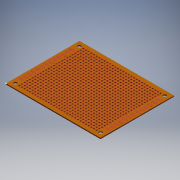
# Autodesk Inventor part: Adafruit_ProtoBoard
Saved by Autodesk Inventor 2018 (Build 220112000, 112)
## iProperties
Created: 2019-08-07
Part Number: Adafruit_ProtoBoard
Material: Generic
Document SubType Name: Modeling
Designer: jhernandez
Density: 1 g/cm^3
Appearance: Copper - Polished
Author: jhernandez
Autodesk Inventor part; units mm, degrees
(part 1 of 4)
ref_plane "YZ Plane" through (0, 0, 0) normal (1, 0, 0) x (0, 1, 0)
ref_plane "XZ Plane" through (0, 0, 0) normal (0, 1, 0) x (-1, 0, 0)
ref_plane "XY Plane" through (0, 0, 0) normal (0, 0, 1) x (1, 0, 0)
sketch "Sketch1" plane through (0, 0, 0) normal (0, 1, 0) x (-1, 0, 0)
  line L0 (0, 0) -> (-90, 0)
  line L1 (-90, 0) -> (-90, -70)
  line L2 (-90, -70) -> (0, -70)
  line L3 (0, -70) -> (0, 0)
  dimension "d0" = 90
  dimension "d1" = 70
  constraints: 8 end point, 2 parallel, 1 horizontal, 1 perpendicular
  measures "d0" distance of L1.end L2.end
  measures "d1" distance of L0.end L1.end
extrude "Extrusion1" add sketch "Sketch1" along normal blind 1
sketch "Sketch2" plane through (0, 1, 0) normal (0, 1, 0) x (1, 0, 0)
  line L0 (0, 0) -> (90, 0) construction
  line L1 (90, 0) -> (90, 70) construction
  line L2 (90, 70) -> (0, 70) construction
  line L3 (0, 70) -> (0, 0) construction
  line L4 (0, 70) -> (0, 0) construction
  line L5 (0, 35) -> (90, 35) construction
  line L6 (90, 70) -> (0, 70) construction
  line L7 (45, 70) -> (45, 0) construction
  circle A0 centre (4.36, 65.48) radius 1.5494
  circle A1 centre (85.64, 65.48) radius 1.5494
  circle A2 centre (4.36, 4.52) radius 1.5494
  circle A3 centre (85.64, 4.52) radius 1.5494
  dimension "d4" = 81.28
  dimension "d5" = 60.96
  dimension "d6" = 3.0988
  constraints: 4 centre point, 4 end point, 4 midpoint, 3 symmetric about line, 3 other
  measures "d4" diameter of A0.centre L7
  measures "d5" diameter of A0.centre L5
  measures "d6" diameter of A0
extrude "Mounting_Holes" cut sketch "Sketch2" against normal up to next
sketch "Sketch5" plane through (0, 1, 0) normal (0, 1, 0) x (1, 0, 0)
  line L0 (90, 70) -> (0, 70) construction
  line L1 (90, 0) -> (90, 70) construction
  line L2 (0, 0) -> (90, 0) construction
  line L3 (0, 70) -> (0, 0) construction
  line L4 (90, 0) -> (90, 70) construction
  line L5 (90, 35) -> (0, 35) construction
  line L6 (45, 70) -> (45, 0) construction
  line L7 (87.4, 35) -> (85.1, 35) construction
  line L8 (87.4, 36.35) -> (85.1, 36.35)
  line L9 (85.1, 33.65) -> (87.4, 33.65)
  arc A0 (87.4, 33.65) -> (87.4, 36.35) centre (87.4, 35) ccw
  arc A1 (85.1, 36.35) -> (85.1, 33.65) centre (85.1, 35) ccw
  arc A2 (87.4, 37.65) -> (87.4, 40.35) centre (87.4, 39) ccw
  line L10 (85.1, 37.65) -> (87.4, 37.65)
  line L11 (87.4, 40.35) -> (85.1, 40.35)
  arc A3 (85.1, 40.35) -> (85.1, 37.65) centre (85.1, 39) ccw
  arc A4 (87.4, 41.65) -> (87.4, 44.35) centre (87.4, 43) ccw
  line L12 (85.1, 41.65) -> (87.4, 41.65)
  line L13 (87.4, 44.35) -> (85.1, 44.35)
  arc A5 (85.1, 44.35) -> (85.1, 41.65) centre (85.1, 43) ccw
  arc A6 (87.4, 45.65) -> (87.4, 48.35) centre (87.4, 47) ccw
  line L14 (85.1, 45.65) -> (87.4, 45.65)
  line L15 (87.4, 48.35) -> (85.1, 48.35)
  arc A7 (85.1, 48.35) -> (85.1, 45.65) centre (85.1, 47) ccw
  arc A8 (87.4, 49.65) -> (87.4, 52.35) centre (87.4, 51) ccw
  line L16 (85.1, 49.65) -> (87.4, 49.65)
  line L17 (87.4, 52.35) -> (85.1, 52.35)
  arc A9 (85.1, 52.35) -> (85.1, 49.65) centre (85.1, 51) ccw
  arc A10 (87.4, 53.65) -> (87.4, 56.35) centre (87.4, 55) ccw
  line L18 (85.1, 53.65) -> (87.4, 53.65)
  line L19 (87.4, 56.35) -> (85.1, 56.35)
  arc A11 (85.1, 56.35) -> (85.1, 53.65) centre (85.1, 55) ccw
  arc A12 (87.4, 57.65) -> (87.4, 60.35) centre (87.4, 59) ccw
  line L20 (85.1, 57.65) -> (87.4, 57.65)
  line L21 (87.4, 60.35) -> (85.1, 60.35)
  arc A13 (85.1, 60.35) -> (85.1, 57.65) centre (85.1, 59) ccw
  arc A14 (87.4, 29.65) -> (87.4, 32.35) centre (87.4, 31) ccw
  line L22 (85.1, 29.65) -> (87.4, 29.65)
  line L23 (87.4, 32.35) -> (85.1, 32.35)
  arc A15 (85.1, 32.35) -> (85.1, 29.65) centre (85.1, 31) ccw
  arc A16 (87.4, 33.65) -> (87.4, 36.35) centre (87.4, 35) ccw
  line L24 (85.1, 33.65) -> (87.4, 33.65)
  line L25 (87.4, 36.35) -> (85.1, 36.35)
  arc A17 (85.1, 36.35) -> (85.1, 33.65) centre (85.1, 35) ccw
  arc A18 (87.4, 37.65) -> (87.4, 40.35) centre (87.4, 39) ccw
  line L26 (85.1, 37.65) -> (87.4, 37.65)
  line L27 (87.4, 40.35) -> (85.1, 40.35)
  arc A19 (85.1, 40.35) -> (85.1, 37.65) centre (85.1, 39) ccw
  arc A20 (87.4, 41.65) -> (87.4, 44.35) centre (87.4, 43) ccw
  line L28 (85.1, 41.65) -> (87.4, 41.65)
  line L29 (87.4, 44.35) -> (85.1, 44.35)
  arc A21 (85.1, 44.35) -> (85.1, 41.65) centre (85.1, 43) ccw
  arc A22 (87.4, 45.65) -> (87.4, 48.35) centre (87.4, 47) ccw
  line L30 (85.1, 45.65) -> (87.4, 45.65)
  line L31 (87.4, 48.35) -> (85.1, 48.35)
  arc A23 (85.1, 48.35) -> (85.1, 45.65) centre (85.1, 47) ccw
  arc A24 (87.4, 49.65) -> (87.4, 52.35) centre (87.4, 51) ccw
  line L32 (85.1, 49.65) -> (87.4, 49.65)
  line L33 (87.4, 52.35) -> (85.1, 52.35)
  arc A25 (85.1, 52.35) -> (85.1, 49.65) centre (85.1, 51) ccw
  arc A26 (87.4, 53.65) -> (87.4, 56.35) centre (87.4, 55) ccw
  line L34 (85.1, 53.65) -> (87.4, 53.65)
  line L35 (87.4, 56.35) -> (85.1, 56.35)
  arc A27 (85.1, 56.35) -> (85.1, 53.65) centre (85.1, 55) ccw
  arc A28 (87.4, 25.65) -> (87.4, 28.35) centre (87.4, 27) ccw
  line L36 (85.1, 25.65) -> (87.4, 25.65)
  line L37 (87.4, 28.35) -> (85.1, 28.35)
  arc A29 (85.1, 28.35) -> (85.1, 25.65) centre (85.1, 27) ccw
  arc A30 (87.4, 29.65) -> (87.4, 32.35) centre (87.4, 31) ccw
  line L38 (85.1, 29.65) -> (87.4, 29.65)
  line L39 (87.4, 32.35) -> (85.1, 32.35)
  arc A31 (85.1, 32.35) -> (85.1, 29.65) centre (85.1, 31) ccw
  arc A32 (87.4, 33.65) -> (87.4, 36.35) centre (87.4, 35) ccw
  line L40 (85.1, 33.65) -> (87.4, 33.65)
  line L41 (87.4, 36.35) -> (85.1, 36.35)
  arc A33 (85.1, 36.35) -> (85.1, 33.65) centre (85.1, 35) ccw
  arc A34 (87.4, 37.65) -> (87.4, 40.35) centre (87.4, 39) ccw
  line L42 (85.1, 37.65) -> (87.4, 37.65)
  line L43 (87.4, 40.35) -> (85.1, 40.35)
  arc A35 (85.1, 40.35) -> (85.1, 37.65) centre (85.1, 39) ccw
  arc A36 (87.4, 41.65) -> (87.4, 44.35) centre (87.4, 43) ccw
  line L44 (85.1, 41.65) -> (87.4, 41.65)
  line L45 (87.4, 44.35) -> (85.1, 44.35)
  arc A37 (85.1, 44.35) -> (85.1, 41.65) centre (85.1, 43) ccw
  arc A38 (87.4, 45.65) -> (87.4, 48.35) centre (87.4, 47) ccw
  line L46 (85.1, 45.65) -> (87.4, 45.65)
  line L47 (87.4, 48.35) -> (85.1, 48.35)
  arc A39 (85.1, 48.35) -> (85.1, 45.65) centre (85.1, 47) ccw
  arc A40 (87.4, 49.65) -> (87.4, 52.35) centre (87.4, 51) ccw
  line L48 (85.1, 49.65) -> (87.4, 49.65)
  line L49 (87.4, 52.35) -> (85.1, 52.35)
  arc A41 (85.1, 52.35) -> (85.1, 49.65) centre (85.1, 51) ccw
  arc A42 (87.4, 21.65) -> (87.4, 24.35) centre (87.4, 23) ccw
  line L50 (85.1, 21.65) -> (87.4, 21.65)
  line L51 (87.4, 24.35) -> (85.1, 24.35)
  arc A43 (85.1, 24.35) -> (85.1, 21.65) centre (85.1, 23) ccw
  arc A44 (87.4, 25.65) -> (87.4, 28.35) centre (87.4, 27) ccw
  line L52 (85.1, 25.65) -> (87.4, 25.65)
  line L53 (87.4, 28.35) -> (85.1, 28.35)
  arc A45 (85.1, 28.35) -> (85.1, 25.65) centre (85.1, 27) ccw
  arc A46 (87.4, 29.65) -> (87.4, 32.35) centre (87.4, 31) ccw
  line L54 (85.1, 29.65) -> (87.4, 29.65)
  line L55 (87.4, 32.35) -> (85.1, 32.35)
  arc A47 (85.1, 32.35) -> (85.1, 29.65) centre (85.1, 31) ccw
  arc A48 (87.4, 33.65) -> (87.4, 36.35) centre (87.4, 35) ccw
  line L56 (85.1, 33.65) -> (87.4, 33.65)
  line L57 (87.4, 36.35) -> (85.1, 36.35)
  arc A49 (85.1, 36.35) -> (85.1, 33.65) centre (85.1, 35) ccw
  arc A50 (87.4, 37.65) -> (87.4, 40.35) centre (87.4, 39) ccw
  line L58 (85.1, 37.65) -> (87.4, 37.65)
  line L59 (87.4, 40.35) -> (85.1, 40.35)
  arc A51 (85.1, 40.35) -> (85.1, 37.65) centre (85.1, 39) ccw
  arc A52 (87.4, 41.65) -> (87.4, 44.35) centre (87.4, 43) ccw
  line L60 (85.1, 41.65) -> (87.4, 41.65)
  line L61 (87.4, 44.35) -> (85.1, 44.35)
  arc A53 (85.1, 44.35) -> (85.1, 41.65) centre (85.1, 43) ccw
  arc A54 (87.4, 45.65) -> (87.4, 48.35) centre (87.4, 47) ccw
  line L62 (85.1, 45.65) -> (87.4, 45.65)
  line L63 (87.4, 48.35) -> (85.1, 48.35)
  arc A55 (85.1, 48.35) -> (85.1, 45.65) centre (85.1, 47) ccw
  arc A56 (87.4, 17.65) -> (87.4, 20.35) centre (87.4, 19) ccw
  line L64 (85.1, 17.65) -> (87.4, 17.65)
  line L65 (87.4, 20.35) -> (85.1, 20.35)
  arc A57 (85.1, 20.35) -> (85.1, 17.65) centre (85.1, 19) ccw
  arc A58 (87.4, 21.65) -> (87.4, 24.35) centre (87.4, 23) ccw
  line L66 (85.1, 21.65) -> (87.4, 21.65)
  line L67 (87.4, 24.35) -> (85.1, 24.35)
  arc A59 (85.1, 24.35) -> (85.1, 21.65) centre (85.1, 23) ccw
  arc A60 (87.4, 25.65) -> (87.4, 28.35) centre (87.4, 27) ccw
  line L68 (85.1, 25.65) -> (87.4, 25.65)
  line L69 (87.4, 28.35) -> (85.1, 28.35)
  arc A61 (85.1, 28.35) -> (85.1, 25.65) centre (85.1, 27) ccw
  arc A62 (87.4, 29.65) -> (87.4, 32.35) centre (87.4, 31) ccw
  line L70 (85.1, 29.65) -> (87.4, 29.65)
  line L71 (87.4, 32.35) -> (85.1, 32.35)
  arc A63 (85.1, 32.35) -> (85.1, 29.65) centre (85.1, 31) ccw
  arc A64 (87.4, 33.65) -> (87.4, 36.35) centre (87.4, 35) ccw
  line L72 (85.1, 33.65) -> (87.4, 33.65)
  line L73 (87.4, 36.35) -> (85.1, 36.35)
  arc A65 (85.1, 36.35) -> (85.1, 33.65) centre (85.1, 35) ccw
  arc A66 (87.4, 37.65) -> (87.4, 40.35) centre (87.4, 39) ccw
  line L74 (85.1, 37.65) -> (87.4, 37.65)
  line L75 (87.4, 40.35) -> (85.1, 40.35)
  arc A67 (85.1, 40.35) -> (85.1, 37.65) centre (85.1, 39) ccw
  arc A68 (87.4, 41.65) -> (87.4, 44.35) centre (87.4, 43) ccw
  line L76 (85.1, 41.65) -> (87.4, 41.65)
  line L77 (87.4, 44.35) -> (85.1, 44.35)
  arc A69 (85.1, 44.35) -> (85.1, 41.65) centre (85.1, 43) ccw
  arc A70 (87.4, 13.65) -> (87.4, 16.35) centre (87.4, 15) ccw
  line L78 (85.1, 13.65) -> (87.4, 13.65)
  line L79 (87.4, 16.35) -> (85.1, 16.35)
  arc A71 (85.1, 16.35) -> (85.1, 13.65) centre (85.1, 15) ccw
  arc A72 (87.4, 17.65) -> (87.4, 20.35) centre (87.4, 19) ccw
  line L80 (85.1, 17.65) -> (87.4, 17.65)
  line L81 (87.4, 20.35) -> (85.1, 20.35)
  arc A73 (85.1, 20.35) -> (85.1, 17.65) centre (85.1, 19) ccw
  arc A74 (87.4, 21.65) -> (87.4, 24.35) centre (87.4, 23) ccw
  line L82 (85.1, 21.65) -> (87.4, 21.65)
  line L83 (87.4, 24.35) -> (85.1, 24.35)
  arc A75 (85.1, 24.35) -> (85.1, 21.65) centre (85.1, 23) ccw
  arc A76 (87.4, 25.65) -> (87.4, 28.35) centre (87.4, 27) ccw
  line L84 (85.1, 25.65) -> (87.4, 25.65)
  line L85 (87.4, 28.35) -> (85.1, 28.35)
  arc A77 (85.1, 28.35) -> (85.1, 25.65) centre (85.1, 27) ccw
  arc A78 (87.4, 29.65) -> (87.4, 32.35) centre (87.4, 31) ccw
  line L86 (85.1, 29.65) -> (87.4, 29.65)
  line L87 (87.4, 32.35) -> (85.1, 32.35)
  arc A79 (85.1, 32.35) -> (85.1, 29.65) centre (85.1, 31) ccw
  arc A80 (87.4, 33.65) -> (87.4, 36.35) centre (87.4, 35) ccw
  line L88 (85.1, 33.65) -> (87.4, 33.65)
  line L89 (87.4, 36.35) -> (85.1, 36.35)
  arc A81 (85.1, 36.35) -> (85.1, 33.65) centre (85.1, 35) ccw
  arc A82 (87.4, 37.65) -> (87.4, 40.35) centre (87.4, 39) ccw
  line L90 (85.1, 37.65) -> (87.4, 37.65)
  line L91 (87.4, 40.35) -> (85.1, 40.35)
  arc A83 (85.1, 40.35) -> (85.1, 37.65) centre (85.1, 39) ccw
  arc A84 (87.4, 9.65) -> (87.4, 12.35) centre (87.4, 11) ccw
  line L92 (85.1, 9.65) -> (87.4, 9.65)
  line L93 (87.4, 12.35) -> (85.1, 12.35)
  arc A85 (85.1, 12.35) -> (85.1, 9.65) centre (85.1, 11) ccw
  arc A86 (87.4, 13.65) -> (87.4, 16.35) centre (87.4, 15) ccw
  line L94 (85.1, 13.65) -> (87.4, 13.65)
  line L95 (87.4, 16.35) -> (85.1, 16.35)
  arc A87 (85.1, 16.35) -> (85.1, 13.65) centre (85.1, 15) ccw
  arc A88 (87.4, 17.65) -> (87.4, 20.35) centre (87.4, 19) ccw
  line L96 (85.1, 17.65) -> (87.4, 17.65)
  line L97 (87.4, 20.35) -> (85.1, 20.35)
  arc A89 (85.1, 20.35) -> (85.1, 17.65) centre (85.1, 19) ccw
  arc A90 (87.4, 21.65) -> (87.4, 24.35) centre (87.4, 23) ccw
  line L98 (85.1, 21.65) -> (87.4, 21.65)
  line L99 (87.4, 24.35) -> (85.1, 24.35)
  arc A91 (85.1, 24.35) -> (85.1, 21.65) centre (85.1, 23) ccw
  arc A92 (87.4, 25.65) -> (87.4, 28.35) centre (87.4, 27) ccw
  line L100 (85.1, 25.65) -> (87.4, 25.65)
  line L101 (87.4, 28.35) -> (85.1, 28.35)
  arc A93 (85.1, 28.35) -> (85.1, 25.65) centre (85.1, 27) ccw
  arc A94 (87.4, 29.65) -> (87.4, 32.35) centre (87.4, 31) ccw
  line L102 (85.1, 29.65) -> (87.4, 29.65)
  line L103 (87.4, 32.35) -> (85.1, 32.35)
  arc A95 (85.1, 32.35) -> (85.1, 29.65) centre (85.1, 31) ccw
  arc A96 (87.4, 33.65) -> (87.4, 36.35) centre (87.4, 35) ccw
  line L104 (85.1, 33.65) -> (87.4, 33.65)
  line L105 (87.4, 36.35) -> (85.1, 36.35)
  arc A97 (85.1, 36.35) -> (85.1, 33.65) centre (85.1, 35) ccw
  line L106 (2.6, 35) -> (4.9, 35) construction
  line L107 (2.6, 36.35) -> (4.9, 36.35)
  line L108 (4.9, 33.65) -> (2.6, 33.65)
  arc A98 (2.6, 36.35) -> (2.6, 33.65) centre (2.6, 35) ccw
  arc A99 (4.9, 33.65) -> (4.9, 36.35) centre (4.9, 35) ccw
  arc A100 (2.6, 40.35) -> (2.6, 37.65) centre (2.6, 39) ccw
  line L109 (4.9, 37.65) -> (2.6, 37.65)
  line L110 (2.6, 40.35) -> (4.9, 40.35)
  arc A101 (4.9, 37.65) -> (4.9, 40.35) centre (4.9, 39) ccw
  arc A102 (2.6, 44.35) -> (2.6, 41.65) centre (2.6, 43) ccw
  line L111 (4.9, 41.65) -> (2.6, 41.65)
  line L112 (2.6, 44.35) -> (4.9, 44.35)
  arc A103 (4.9, 41.65) -> (4.9, 44.35) centre (4.9, 43) ccw
  arc A104 (2.6, 48.35) -> (2.6, 45.65) centre (2.6, 47) ccw
  line L113 (4.9, 45.65) -> (2.6, 45.65)
  line L114 (2.6, 48.35) -> (4.9, 48.35)
  arc A105 (4.9, 45.65) -> (4.9, 48.35) centre (4.9, 47) ccw
  arc A106 (2.6, 52.35) -> (2.6, 49.65) centre (2.6, 51) ccw
  line L115 (4.9, 49.65) -> (2.6, 49.65)
  line L116 (2.6, 52.35) -> (4.9, 52.35)
  arc A107 (4.9, 49.65) -> (4.9, 52.35) centre (4.9, 51) ccw
  arc A108 (2.6, 56.35) -> (2.6, 53.65) centre (2.6, 55) ccw
  line L117 (4.9, 53.65) -> (2.6, 53.65)
  line L118 (2.6, 56.35) -> (4.9, 56.35)
  arc A109 (4.9, 53.65) -> (4.9, 56.35) centre (4.9, 55) ccw
  arc A110 (2.6, 60.35) -> (2.6, 57.65) centre (2.6, 59) ccw
  line L119 (4.9, 57.65) -> (2.6, 57.65)
  line L120 (2.6, 60.35) -> (4.9, 60.35)
  arc A111 (4.9, 57.65) -> (4.9, 60.35) centre (4.9, 59) ccw
  arc A112 (2.6, 32.35) -> (2.6, 29.65) centre (2.6, 31) ccw
  line L121 (4.9, 29.65) -> (2.6, 29.65)
  line L122 (2.6, 32.35) -> (4.9, 32.35)
  arc A113 (4.9, 29.65) -> (4.9, 32.35) centre (4.9, 31) ccw
  arc A114 (2.6, 36.35) -> (2.6, 33.65) centre (2.6, 35) ccw
  line L123 (4.9, 33.65) -> (2.6, 33.65)
  line L124 (2.6, 36.35) -> (4.9, 36.35)
  arc A115 (4.9, 33.65) -> (4.9, 36.35) centre (4.9, 35) ccw
  arc A116 (2.6, 40.35) -> (2.6, 37.65) centre (2.6, 39) ccw
  line L125 (4.9, 37.65) -> (2.6, 37.65)
  line L126 (2.6, 40.35) -> (4.9, 40.35)
  arc A117 (4.9, 37.65) -> (4.9, 40.35) centre (4.9, 39) ccw
  arc A118 (2.6, 44.35) -> (2.6, 41.65) centre (2.6, 43) ccw
  line L127 (4.9, 41.65) -> (2.6, 41.65)
  line L128 (2.6, 44.35) -> (4.9, 44.35)
  arc A119 (4.9, 41.65) -> (4.9, 44.35) centre (4.9, 43) ccw
  arc A120 (2.6, 48.35) -> (2.6, 45.65) centre (2.6, 47) ccw
  line L129 (4.9, 45.65) -> (2.6, 45.65)
  line L130 (2.6, 48.35) -> (4.9, 48.35)
  arc A121 (4.9, 45.65) -> (4.9, 48.35) centre (4.9, 47) ccw
  arc A122 (2.6, 52.35) -> (2.6, 49.65) centre (2.6, 51) ccw
  line L131 (4.9, 49.65) -> (2.6, 49.65)
  line L132 (2.6, 52.35) -> (4.9, 52.35)
  arc A123 (4.9, 49.65) -> (4.9, 52.35) centre (4.9, 51) ccw
  arc A124 (2.6, 56.35) -> (2.6, 53.65) centre (2.6, 55) ccw
  line L133 (4.9, 53.65) -> (2.6, 53.65)
  line L134 (2.6, 56.35) -> (4.9, 56.35)
  arc A125 (4.9, 53.65) -> (4.9, 56.35) centre (4.9, 55) ccw
  arc A126 (2.6, 28.35) -> (2.6, 25.65) centre (2.6, 27) ccw
  line L135 (4.9, 25.65) -> (2.6, 25.65)
  line L136 (2.6, 28.35) -> (4.9, 28.35)
  arc A127 (4.9, 25.65) -> (4.9, 28.35) centre (4.9, 27) ccw
  arc A128 (2.6, 32.35) -> (2.6, 29.65) centre (2.6, 31) ccw
  line L137 (4.9, 29.65) -> (2.6, 29.65)
  line L138 (2.6, 32.35) -> (4.9, 32.35)
  arc A129 (4.9, 29.65) -> (4.9, 32.35) centre (4.9, 31) ccw
  arc A130 (2.6, 36.35) -> (2.6, 33.65) centre (2.6, 35) ccw
  line L139 (4.9, 33.65) -> (2.6, 33.65)
  line L140 (2.6, 36.35) -> (4.9, 36.35)
  arc A131 (4.9, 33.65) -> (4.9, 36.35) centre (4.9, 35) ccw
  arc A132 (2.6, 40.35) -> (2.6, 37.65) centre (2.6, 39) ccw
  line L141 (4.9, 37.65) -> (2.6, 37.65)
  line L142 (2.6, 40.35) -> (4.9, 40.35)
  arc A133 (4.9, 37.65) -> (4.9, 40.35) centre (4.9, 39) ccw
  arc A134 (2.6, 44.35) -> (2.6, 41.65) centre (2.6, 43) ccw
  line L143 (4.9, 41.65) -> (2.6, 41.65)
  line L144 (2.6, 44.35) -> (4.9, 44.35)
  arc A135 (4.9, 41.65) -> (4.9, 44.35) centre (4.9, 43) ccw
  arc A136 (2.6, 48.35) -> (2.6, 45.65) centre (2.6, 47) ccw
  line L145 (4.9, 45.65) -> (2.6, 45.65)
  line L146 (2.6, 48.35) -> (4.9, 48.35)
  arc A137 (4.9, 45.65) -> (4.9, 48.35) centre (4.9, 47) ccw
  arc A138 (2.6, 52.35) -> (2.6, 49.65) centre (2.6, 51) ccw
  line L147 (4.9, 49.65) -> (2.6, 49.65)
  line L148 (2.6, 52.35) -> (4.9, 52.35)
  arc A139 (4.9, 49.65) -> (4.9, 52.35) centre (4.9, 51) ccw
  arc A140 (2.6, 24.35) -> (2.6, 21.65) centre (2.6, 23) ccw
  line L149 (4.9, 21.65) -> (2.6, 21.65)
  line L150 (2.6, 24.35) -> (4.9, 24.35)
  arc A141 (4.9, 21.65) -> (4.9, 24.35) centre (4.9, 23) ccw
  arc A142 (2.6, 28.35) -> (2.6, 25.65) centre (2.6, 27) ccw
  line L151 (4.9, 25.65) -> (2.6, 25.65)
  line L152 (2.6, 28.35) -> (4.9, 28.35)
  arc A143 (4.9, 25.65) -> (4.9, 28.35) centre (4.9, 27) ccw
  arc A144 (2.6, 32.35) -> (2.6, 29.65) centre (2.6, 31) ccw
  line L153 (4.9, 29.65) -> (2.6, 29.65)
  line L154 (2.6, 32.35) -> (4.9, 32.35)
  arc A145 (4.9, 29.65) -> (4.9, 32.35) centre (4.9, 31) ccw
  arc A146 (2.6, 36.35) -> (2.6, 33.65) centre (2.6, 35) ccw
  line L155 (4.9, 33.65) -> (2.6, 33.65)
  line L156 (2.6, 36.35) -> (4.9, 36.35)
  arc A147 (4.9, 33.65) -> (4.9, 36.35) centre (4.9, 35) ccw
  arc A148 (2.6, 40.35) -> (2.6, 37.65) centre (2.6, 39) ccw
  line L157 (4.9, 37.65) -> (2.6, 37.65)
  line L158 (2.6, 40.35) -> (4.9, 40.35)
  arc A149 (4.9, 37.65) -> (4.9, 40.35) centre (4.9, 39) ccw
  arc A150 (2.6, 44.35) -> (2.6, 41.65) centre (2.6, 43) ccw
  line L159 (4.9, 41.65) -> (2.6, 41.65)
  line L160 (2.6, 44.35) -> (4.9, 44.35)
  arc A151 (4.9, 41.65) -> (4.9, 44.35) centre (4.9, 43) ccw
  arc A152 (2.6, 48.35) -> (2.6, 45.65) centre (2.6, 47) ccw
  line L161 (4.9, 45.65) -> (2.6, 45.65)
  line L162 (2.6, 48.35) -> (4.9, 48.35)
  arc A153 (4.9, 45.65) -> (4.9, 48.35) centre (4.9, 47) ccw
  arc A154 (2.6, 20.35) -> (2.6, 17.65) centre (2.6, 19) ccw
  line L163 (4.9, 17.65) -> (2.6, 17.65)
  line L164 (2.6, 20.35) -> (4.9, 20.35)
  arc A155 (4.9, 17.65) -> (4.9, 20.35) centre (4.9, 19) ccw
  arc A156 (2.6, 24.35) -> (2.6, 21.65) centre (2.6, 23) ccw
  line L165 (4.9, 21.65) -> (2.6, 21.65)
  line L166 (2.6, 24.35) -> (4.9, 24.35)
  arc A157 (4.9, 21.65) -> (4.9, 24.35) centre (4.9, 23) ccw
  arc A158 (2.6, 28.35) -> (2.6, 25.65) centre (2.6, 27) ccw
  line L167 (4.9, 25.65) -> (2.6, 25.65)
  line L168 (2.6, 28.35) -> (4.9, 28.35)
  arc A159 (4.9, 25.65) -> (4.9, 28.35) centre (4.9, 27) ccw
  arc A160 (2.6, 32.35) -> (2.6, 29.65) centre (2.6, 31) ccw
  line L169 (4.9, 29.65) -> (2.6, 29.65)
  line L170 (2.6, 32.35) -> (4.9, 32.35)
  arc A161 (4.9, 29.65) -> (4.9, 32.35) centre (4.9, 31) ccw
  arc A162 (2.6, 36.35) -> (2.6, 33.65) centre (2.6, 35) ccw
  line L171 (4.9, 33.65) -> (2.6, 33.65)
  line L172 (2.6, 36.35) -> (4.9, 36.35)
  arc A163 (4.9, 33.65) -> (4.9, 36.35) centre (4.9, 35) ccw
  arc A164 (2.6, 40.35) -> (2.6, 37.65) centre (2.6, 39) ccw
  line L173 (4.9, 37.65) -> (2.6, 37.65)
  line L174 (2.6, 40.35) -> (4.9, 40.35)
  arc A165 (4.9, 37.65) -> (4.9, 40.35) centre (4.9, 39) ccw
  arc A166 (2.6, 44.35) -> (2.6, 41.65) centre (2.6, 43) ccw
  line L175 (4.9, 41.65) -> (2.6, 41.65)
  line L176 (2.6, 44.35) -> (4.9, 44.35)
  arc A167 (4.9, 41.65) -> (4.9, 44.35) centre (4.9, 43) ccw
  arc A168 (2.6, 16.35) -> (2.6, 13.65) centre (2.6, 15) ccw
  line L177 (4.9, 13.65) -> (2.6, 13.65)
  line L178 (2.6, 16.35) -> (4.9, 16.35)
  arc A169 (4.9, 13.65) -> (4.9, 16.35) centre (4.9, 15) ccw
  arc A170 (2.6, 20.35) -> (2.6, 17.65) centre (2.6, 19) ccw
  line L179 (4.9, 17.65) -> (2.6, 17.65)
  line L180 (2.6, 20.35) -> (4.9, 20.35)
  arc A171 (4.9, 17.65) -> (4.9, 20.35) centre (4.9, 19) ccw
  arc A172 (2.6, 24.35) -> (2.6, 21.65) centre (2.6, 23) ccw
  line L181 (4.9, 21.65) -> (2.6, 21.65)
  line L182 (2.6, 24.35) -> (4.9, 24.35)
  arc A173 (4.9, 21.65) -> (4.9, 24.35) centre (4.9, 23) ccw
  arc A174 (2.6, 28.35) -> (2.6, 25.65) centre (2.6, 27) ccw
  line L183 (4.9, 25.65) -> (2.6, 25.65)
  line L184 (2.6, 28.35) -> (4.9, 28.35)
  arc A175 (4.9, 25.65) -> (4.9, 28.35) centre (4.9, 27) ccw
  arc A176 (2.6, 32.35) -> (2.6, 29.65) centre (2.6, 31) ccw
  line L185 (4.9, 29.65) -> (2.6, 29.65)
  line L186 (2.6, 32.35) -> (4.9, 32.35)
  arc A177 (4.9, 29.65) -> (4.9, 32.35) centre (4.9, 31) ccw
  arc A178 (2.6, 36.35) -> (2.6, 33.65) centre (2.6, 35) ccw
  line L187 (4.9, 33.65) -> (2.6, 33.65)
  line L188 (2.6, 36.35) -> (4.9, 36.35)
  arc A179 (4.9, 33.65) -> (4.9, 36.35) centre (4.9, 35) ccw
  arc A180 (2.6, 40.35) -> (2.6, 37.65) centre (2.6, 39) ccw
  line L189 (4.9, 37.65) -> (2.6, 37.65)
  line L190 (2.6, 40.35) -> (4.9, 40.35)
  arc A181 (4.9, 37.65) -> (4.9, 40.35) centre (4.9, 39) ccw
  arc A182 (2.6, 12.35) -> (2.6, 9.65) centre (2.6, 11) ccw
  line L191 (4.9, 9.65) -> (2.6, 9.65)
  line L192 (2.6, 12.35) -> (4.9, 12.35)
  arc A183 (4.9, 9.65) -> (4.9, 12.35) centre (4.9, 11) ccw
  arc A184 (2.6, 16.35) -> (2.6, 13.65) centre (2.6, 15) ccw
  line L193 (4.9, 13.65) -> (2.6, 13.65)
  line L194 (2.6, 16.35) -> (4.9, 16.35)
  arc A185 (4.9, 13.65) -> (4.9, 16.35) centre (4.9, 15) ccw
  arc A186 (2.6, 20.35) -> (2.6, 17.65) centre (2.6, 19) ccw
  line L195 (4.9, 17.65) -> (2.6, 17.65)
  line L196 (2.6, 20.35) -> (4.9, 20.35)
  arc A187 (4.9, 17.65) -> (4.9, 20.35) centre (4.9, 19) ccw
  arc A188 (2.6, 24.35) -> (2.6, 21.65) centre (2.6, 23) ccw
  line L197 (4.9, 21.65) -> (2.6, 21.65)
  line L198 (2.6, 24.35) -> (4.9, 24.35)
  arc A189 (4.9, 21.65) -> (4.9, 24.35) centre (4.9, 23) ccw
  arc A190 (2.6, 28.35) -> (2.6, 25.65) centre (2.6, 27) ccw
  line L199 (4.9, 25.65) -> (2.6, 25.65)
  line L200 (2.6, 28.35) -> (4.9, 28.35)
  arc A191 (4.9, 25.65) -> (4.9, 28.35) centre (4.9, 27) ccw
  arc A192 (2.6, 32.35) -> (2.6, 29.65) centre (2.6, 31) ccw
  line L201 (4.9, 29.65) -> (2.6, 29.65)
  line L202 (2.6, 32.35) -> (4.9, 32.35)
  arc A193 (4.9, 29.65) -> (4.9, 32.35) centre (4.9, 31) ccw
  arc A194 (2.6, 36.35) -> (2.6, 33.65) centre (2.6, 35) ccw
  line L203 (4.9, 33.65) -> (2.6, 33.65)
  line L204 (2.6, 36.35) -> (4.9, 36.35)
  arc A195 (4.9, 33.65) -> (4.9, 36.35) centre (4.9, 35) ccw
  point P0 (86.25, 35)
  point P1 (3.75, 35)
  dimension "d31" = 2.7
  dimension "d32" = 5
  dimension "d35" = 4
  dimension "d38" = 4
  dimension "d41" = 2.6
  dimension "d42" = 1.35
  constraints: 404 end point, 392 point on circle, 295 symmetric about line, 196 centre point, 5 midpoint, 4 tangent, 2 point on line, 2 vertical, 1 parallel, 578 other
  measures "d31" distance between parallel lines of L9 L8
  measures "d35" distance of L7.start A2.centre
  measures "d38" distance of L7.start A14.centre
  measures "d41" distance from line of L1 L7.start
  measures "d42" radius of A28
extrude "In_Out_Pads" add sketch "Sketch5" along normal blind 0.05
sketch "Sketch3" plane through (0, 1, 0) normal (0, 1, 0) x (1, 0, 0)
  circle A0 centre (8.17, 65.48) radius 1.125
  circle A1 centre (4.36, 4.52) radius 1.5494 construction
  circle A2 centre (4.36, 65.48) radius 1.5494 construction
  circle A3 centre (85.64, 65.48) radius 1.5494 construction
  circle A4 centre (85.64, 4.52) radius 1.5494 construction
  line L0 (0, 0) -> (90, 0) construction
  line L1 (90, 0) -> (90, 70) construction
  line L2 (90, 70) -> (0, 70) construction
  line L3 (0, 70) -> (0, 0) construction
  circle A5 centre (10.71, 65.48) radius 1.125
  circle A6 centre (13.25, 65.48) radius 1.125
  circle A7 centre (15.79, 65.48) radius 1.125
  circle A8 centre (18.33, 65.48) radius 1.125
  circle A9 centre (20.87, 65.48) radius 1.125
  circle A10 centre (23.41, 65.48) radius 1.125
  circle A11 centre (25.95, 65.48) radius 1.125
  circle A12 centre (28.49, 65.48) radius 1.125
  circle A13 centre (31.03, 65.48) radius 1.125
  circle A14 centre (33.57, 65.48) radius 1.125
  circle A15 centre (36.11, 65.48) radius 1.125
  circle A16 centre (38.65, 65.48) radius 1.125
  circle A17 centre (41.19, 65.48) radius 1.125
  circle A18 centre (43.73, 65.48) radius 1.125
  circle A19 centre (46.27, 65.48) radius 1.125
  circle A20 centre (48.81, 65.48) radius 1.125
  circle A21 centre (51.35, 65.48) radius 1.125
  circle A22 centre (53.89, 65.48) radius 1.125
  circle A23 centre (56.43, 65.48) radius 1.125
  circle A24 centre (58.97, 65.48) radius 1.125
  circle A25 centre (61.51, 65.48) radius 1.125
  circle A26 centre (64.05, 65.48) radius 1.125
  circle A27 centre (66.59, 65.48) radius 1.125
  circle A28 centre (69.13, 65.48) radius 1.125
  circle A29 centre (71.67, 65.48) radius 1.125
  circle A30 centre (74.21, 65.48) radius 1.125
  circle A31 centre (76.75, 65.48) radius 1.125
  circle A32 centre (79.29, 65.48) radius 1.125
  circle A33 centre (81.83, 65.48) radius 1.125
  circle A34 centre (8.17, 62.94) radius 1.125
  circle A35 centre (10.71, 62.94) radius 1.125
  circle A36 centre (13.25, 62.94) radius 1.125
  circle A37 centre (15.79, 62.94) radius 1.125
  circle A38 centre (18.33, 62.94) radius 1.125
  circle A39 centre (20.87, 62.94) radius 1.125
  circle A40 centre (23.41, 62.94) radius 1.125
  circle A41 centre (25.95, 62.94) radius 1.125
  circle A42 centre (28.49, 62.94) radius 1.125
  circle A43 centre (31.03, 62.94) radius 1.125
  circle A44 centre (33.57, 62.94) radius 1.125
  circle A45 centre (36.11, 62.94) radius 1.125
  circle A46 centre (38.65, 62.94) radius 1.125
  circle A47 centre (41.19, 62.94) radius 1.125
  circle A48 centre (43.73, 62.94) radius 1.125
  circle A49 centre (46.27, 62.94) radius 1.125
  circle A50 centre (48.81, 62.94) radius 1.125
  circle A51 centre (51.35, 62.94) radius 1.125
  circle A52 centre (53.89, 62.94) radius 1.125
  circle A53 centre (56.43, 62.94) radius 1.125
  circle A54 centre (58.97, 62.94) radius 1.125
  circle A55 centre (61.51, 62.94) radius 1.125
  circle A56 centre (64.05, 62.94) radius 1.125
  circle A57 centre (66.59, 62.94) radius 1.125
  circle A58 centre (69.13, 62.94) radius 1.125
  circle A59 centre (71.67, 62.94) radius 1.125
  circle A60 centre (74.21, 62.94) radius 1.125
  circle A61 centre (76.75, 62.94) radius 1.125
  circle A62 centre (79.29, 62.94) radius 1.125
  circle A63 centre (81.83, 62.94) radius 1.125
  circle A64 centre (8.17, 60.4) radius 1.125
  circle A65 centre (10.71, 60.4) radius 1.125
  circle A66 centre (13.25, 60.4) radius 1.125
  circle A67 centre (15.79, 60.4) radius 1.125
  circle A68 centre (18.33, 60.4) radius 1.125
  circle A69 centre (20.87, 60.4) radius 1.125
  circle A70 centre (23.41, 60.4) radius 1.125
  circle A71 centre (25.95, 60.4) radius 1.125
  circle A72 centre (28.49, 60.4) radius 1.125
  circle A73 centre (31.03, 60.4) radius 1.125
  circle A74 centre (33.57, 60.4) radius 1.125
  circle A75 centre (36.11, 60.4) radius 1.125
  circle A76 centre (38.65, 60.4) radius 1.125
  circle A77 centre (41.19, 60.4) radius 1.125
  circle A78 centre (43.73, 60.4) radius 1.125
  circle A79 centre (46.27, 60.4) radius 1.125
  circle A80 centre (48.81, 60.4) radius 1.125
  circle A81 centre (51.35, 60.4) radius 1.125
  circle A82 centre (53.89, 60.4) radius 1.125
  circle A83 centre (56.43, 60.4) radius 1.125
  circle A84 centre (58.97, 60.4) radius 1.125
  circle A85 centre (61.51, 60.4) radius 1.125
  circle A86 centre (64.05, 60.4) radius 1.125
  circle A87 centre (66.59, 60.4) radius 1.125
  circle A88 centre (69.13, 60.4) radius 1.125
  circle A89 centre (71.67, 60.4) radius 1.125
  circle A90 centre (74.21, 60.4) radius 1.125
  circle A91 centre (76.75, 60.4) radius 1.125
  circle A92 centre (79.29, 60.4) radius 1.125
  circle A93 centre (81.83, 60.4) radius 1.125
  circle A94 centre (8.17, 57.86) radius 1.125
  circle A95 centre (10.71, 57.86) radius 1.125
  circle A96 centre (13.25, 57.86) radius 1.125
  circle A97 centre (15.79, 57.86) radius 1.125
  circle A98 centre (18.33, 57.86) radius 1.125
  circle A99 centre (20.87, 57.86) radius 1.125
  circle A100 centre (23.41, 57.86) radius 1.125
  circle A101 centre (25.95, 57.86) radius 1.125
  circle A102 centre (28.49, 57.86) radius 1.125
  circle A103 centre (31.03, 57.86) radius 1.125
  circle A104 centre (33.57, 57.86) radius 1.125
  circle A105 centre (36.11, 57.86) radius 1.125
  circle A106 centre (38.65, 57.86) radius 1.125
  circle A107 centre (41.19, 57.86) radius 1.125
  circle A108 centre (43.73, 57.86) radius 1.125
  circle A109 centre (46.27, 57.86) radius 1.125
  circle A110 centre (48.81, 57.86) radius 1.125
  circle A111 centre (51.35, 57.86) radius 1.125
  circle A112 centre (53.89, 57.86) radius 1.125
  circle A113 centre (56.43, 57.86) radius 1.125
  circle A114 centre (58.97, 57.86) radius 1.125
  circle A115 centre (61.51, 57.86) radius 1.125
  circle A116 centre (64.05, 57.86) radius 1.125
  circle A117 centre (66.59, 57.86) radius 1.125
  circle A118 centre (69.13, 57.86) radius 1.125
  circle A119 centre (71.67, 57.86) radius 1.125
  circle A120 centre (74.21, 57.86) radius 1.125
  circle A121 centre (76.75, 57.86) radius 1.125
  circle A122 centre (79.29, 57.86) radius 1.125
  circle A123 centre (81.83, 57.86) radius 1.125
  circle A124 centre (8.17, 55.32) radius 1.125
  circle A125 centre (10.71, 55.32) radius 1.125
  circle A126 centre (13.25, 55.32) radius 1.125
  circle A127 centre (15.79, 55.32) radius 1.125
  circle A128 centre (18.33, 55.32) radius 1.125
  circle A129 centre (20.87, 55.32) radius 1.125
  circle A130 centre (23.41, 55.32) radius 1.125
  circle A131 centre (25.95, 55.32) radius 1.125
  circle A132 centre (28.49, 55.32) radius 1.125
  circle A133 centre (31.03, 55.32) radius 1.125
  circle A134 centre (33.57, 55.32) radius 1.125
  circle A135 centre (36.11, 55.32) radius 1.125
  circle A136 centre (38.65, 55.32) radius 1.125
  circle A137 centre (41.19, 55.32) radius 1.125
  circle A138 centre (43.73, 55.32) radius 1.125
  circle A139 centre (46.27, 55.32) radius 1.125
  circle A140 centre (48.81, 55.32) radius 1.125
  circle A141 centre (51.35, 55.32) radius 1.125
  circle A142 centre (53.89, 55.32) radius 1.125
  circle A143 centre (56.43, 55.32) radius 1.125
  circle A144 centre (58.97, 55.32) radius 1.125
  circle A145 centre (61.51, 55.32) radius 1.125
  circle A146 centre (64.05, 55.32) radius 1.125
  circle A147 centre (66.59, 55.32) radius 1.125
  circle A148 centre (69.13, 55.32) radius 1.125
  circle A149 centre (71.67, 55.32) radius 1.125
  circle A150 centre (74.21, 55.32) radius 1.125
  circle A151 centre (76.75, 55.32) radius 1.125
  circle A152 centre (79.29, 55.32) radius 1.125
  circle A153 centre (81.83, 55.32) radius 1.125
  circle A154 centre (8.17, 52.78) radius 1.125
  circle A155 centre (10.71, 52.78) radius 1.125
  circle A156 centre (13.25, 52.78) radius 1.125
  circle A157 centre (15.79, 52.78) radius 1.125
  circle A158 centre (18.33, 52.78) radius 1.125
  circle A159 centre (20.87, 52.78) radius 1.125
  circle A160 centre (23.41, 52.78) radius 1.125
  circle A161 centre (25.95, 52.78) radius 1.125
  circle A162 centre (28.49, 52.78) radius 1.125
  circle A163 centre (31.03, 52.78) radius 1.125
  circle A164 centre (33.57, 52.78) radius 1.125
  circle A165 centre (36.11, 52.78) radius 1.125
  circle A166 centre (38.65, 52.78) radius 1.125
  circle A167 centre (41.19, 52.78) radius 1.125
  circle A168 centre (43.73, 52.78) radius 1.125
  circle A169 centre (46.27, 52.78) radius 1.125
  circle A170 centre (48.81, 52.78) radius 1.125
  circle A171 centre (51.35, 52.78) radius 1.125
  circle A172 centre (53.89, 52.78) radius 1.125
  circle A173 centre (56.43, 52.78) radius 1.125
  circle A174 centre (58.97, 52.78) radius 1.125
  circle A175 centre (61.51, 52.78) radius 1.125
  circle A176 centre (64.05, 52.78) radius 1.125
  circle A177 centre (66.59, 52.78) radius 1.125
  circle A178 centre (69.13, 52.78) radius 1.125
  circle A179 centre (71.67, 52.78) radius 1.125
  circle A180 centre (74.21, 52.78) radius 1.125
  circle A181 centre (76.75, 52.78) radius 1.125
  circle A182 centre (79.29, 52.78) radius 1.125
  circle A183 centre (81.83, 52.78) radius 1.125
  circle A184 centre (8.17, 50.24) radius 1.125
  circle A185 centre (10.71, 50.24) radius 1.125
  circle A186 centre (13.25, 50.24) radius 1.125
  circle A187 centre (15.79, 50.24) radius 1.125
  circle A188 centre (18.33, 50.24) radius 1.125
  circle A189 centre (20.87, 50.24) radius 1.125
  circle A190 centre (23.41, 50.24) radius 1.125
  circle A191 centre (25.95, 50.24) radius 1.125
  circle A192 centre (28.49, 50.24) radius 1.125
  circle A193 centre (31.03, 50.24) radius 1.125
  circle A194 centre (33.57, 50.24) radius 1.125
  circle A195 centre (36.11, 50.24) radius 1.125
  circle A196 centre (38.65, 50.24) radius 1.125
  circle A197 centre (41.19, 50.24) radius 1.125
  circle A198 centre (43.73, 50.24) radius 1.125
  circle A199 centre (46.27, 50.24) radius 1.125
  circle A200 centre (48.81, 50.24) radius 1.125
  circle A201 centre (51.35, 50.24) radius 1.125
  circle A202 centre (53.89, 50.24) radius 1.125
  circle A203 centre (56.43, 50.24) radius 1.125
  circle A204 centre (58.97, 50.24) radius 1.125
  circle A205 centre (61.51, 50.24) radius 1.125
  circle A206 centre (64.05, 50.24) radius 1.125
  circle A207 centre (66.59, 50.24) radius 1.125
  circle A208 centre (69.13, 50.24) radius 1.125
  circle A209 centre (71.67, 50.24) radius 1.125
  circle A210 centre (74.21, 50.24) radius 1.125
  circle A211 centre (76.75, 50.24) radius 1.125
  circle A212 centre (79.29, 50.24) radius 1.125
  circle A213 centre (81.83, 50.24) radius 1.125
  circle A214 centre (8.17, 47.7) radius 1.125
  circle A215 centre (10.71, 47.7) radius 1.125
  circle A216 centre (13.25, 47.7) radius 1.125
  circle A217 centre (15.79, 47.7) radius 1.125
  circle A218 centre (18.33, 47.7) radius 1.125
  circle A219 centre (20.87, 47.7) radius 1.125
  circle A220 centre (23.41, 47.7) radius 1.125
  circle A221 centre (25.95, 47.7) radius 1.125
  circle A222 centre (28.49, 47.7) radius 1.125
  circle A223 centre (31.03, 47.7) radius 1.125
  circle A224 centre (33.57, 47.7) radius 1.125
  circle A225 centre (36.11, 47.7) radius 1.125
  circle A226 centre (38.65, 47.7) radius 1.125
  circle A227 centre (41.19, 47.7) radius 1.125
  circle A228 centre (43.73, 47.7) radius 1.125
  circle A229 centre (46.27, 47.7) radius 1.125
  circle A230 centre (48.81, 47.7) radius 1.125
  circle A231 centre (51.35, 47.7) radius 1.125
  circle A232 centre (53.89, 47.7) radius 1.125
  circle A233 centre (56.43, 47.7) radius 1.125
  circle A234 centre (58.97, 47.7) radius 1.125
  circle A235 centre (61.51, 47.7) radius 1.125
  circle A236 centre (64.05, 47.7) radius 1.125
  circle A237 centre (66.59, 47.7) radius 1.125
  circle A238 centre (69.13, 47.7) radius 1.125
  circle A239 centre (71.67, 47.7) radius 1.125
  circle A240 centre (74.21, 47.7) radius 1.125
  circle A241 centre (76.75, 47.7) radius 1.125
  circle A242 centre (79.29, 47.7) radius 1.125
  circle A243 centre (81.83, 47.7) radius 1.125
  circle A244 centre (8.17, 45.16) radius 1.125
  circle A245 centre (10.71, 45.16) radius 1.125
  circle A246 centre (13.25, 45.16) radius 1.125
  circle A247 centre (15.79, 45.16) radius 1.125
  circle A248 centre (18.33, 45.16) radius 1.125
  circle A249 centre (20.87, 45.16) radius 1.125
  circle A250 centre (23.41, 45.16) radius 1.125
  circle A251 centre (25.95, 45.16) radius 1.125
  circle A252 centre (28.49, 45.16) radius 1.125
  circle A253 centre (31.03, 45.16) radius 1.125
  circle A254 centre (33.57, 45.16) radius 1.125
  circle A255 centre (36.11, 45.16) radius 1.125
  circle A256 centre (38.65, 45.16) radius 1.125
  circle A257 centre (41.19, 45.16) radius 1.125
  circle A258 centre (43.73, 45.16) radius 1.125
  circle A259 centre (46.27, 45.16) radius 1.125
  circle A260 centre (48.81, 45.16) radius 1.125
  circle A261 centre (51.35, 45.16) radius 1.125
  circle A262 centre (53.89, 45.16) radius 1.125
  circle A263 centre (56.43, 45.16) radius 1.125
  circle A264 centre (58.97, 45.16) radius 1.125
  circle A265 centre (61.51, 45.16) radius 1.125
  circle A266 centre (64.05, 45.16) radius 1.125
  circle A267 centre (66.59, 45.16) radius 1.125
  circle A268 centre (69.13, 45.16) radius 1.125
  circle A269 centre (71.67, 45.16) radius 1.125
  circle A270 centre (74.21, 45.16) radius 1.125
  circle A271 centre (76.75, 45.16) radius 1.125
  circle A272 centre (79.29, 45.16) radius 1.125
  circle A273 centre (81.83, 45.16) radius 1.125
  circle A274 centre (8.17, 42.62) radius 1.125
  circle A275 centre (10.71, 42.62) radius 1.125
  circle A276 centre (13.25, 42.62) radius 1.125
  circle A277 centre (15.79, 42.62) radius 1.125
  circle A278 centre (18.33, 42.62) radius 1.125
  circle A279 centre (20.87, 42.62) radius 1.125
  circle A280 centre (23.41, 42.62) radius 1.125
  circle A281 centre (25.95, 42.62) radius 1.125
  circle A282 centre (28.49, 42.62) radius 1.125
  circle A283 centre (31.03, 42.62) radius 1.125
  circle A284 centre (33.57, 42.62) radius 1.125
  circle A285 centre (36.11, 42.62) radius 1.125
  circle A286 centre (38.65, 42.62) radius 1.125
  circle A287 centre (41.19, 42.62) radius 1.125
  circle A288 centre (43.73, 42.62) radius 1.125
  circle A289 centre (46.27, 42.62) radius 1.125
  circle A290 centre (48.81, 42.62) radius 1.125
  circle A291 centre (51.35, 42.62) radius 1.125
  circle A292 centre (53.89, 42.62) radius 1.125
  circle A293 centre (56.43, 42.62) radius 1.125
  circle A294 centre (58.97, 42.62) radius 1.125
  circle A295 centre (61.51, 42.62) radius 1.125
  circle A296 centre (64.05, 42.62) radius 1.125
  circle A297 centre (66.59, 42.62) radius 1.125
  circle A298 centre (69.13, 42.62) radius 1.125
  circle A299 centre (71.67, 42.62) radius 1.125
  circle A300 centre (74.21, 42.62) radius 1.125
  circle A301 centre (76.75, 42.62) radius 1.125
  circle A302 centre (79.29, 42.62) radius 1.125
  circle A303 centre (81.83, 42.62) radius 1.125
  circle A304 centre (8.17, 40.08) radius 1.125
  circle A305 centre (10.71, 40.08) radius 1.125
  circle A306 centre (13.25, 40.08) radius 1.125
  circle A307 centre (15.79, 40.08) radius 1.125
  circle A308 centre (18.33, 40.08) radius 1.125
  circle A309 centre (20.87, 40.08) radius 1.125
  circle A310 centre (23.41, 40.08) radius 1.125
  circle A311 centre (25.95, 40.08) radius 1.125
  circle A312 centre (28.49, 40.08) radius 1.125
  circle A313 centre (31.03, 40.08) radius 1.125
  circle A314 centre (33.57, 40.08) radius 1.125
  circle A315 centre (36.11, 40.08) radius 1.125
  circle A316 centre (38.65, 40.08) radius 1.125
  circle A317 centre (41.19, 40.08) radius 1.125
  circle A318 centre (43.73, 40.08) radius 1.125
  circle A319 centre (46.27, 40.08) radius 1.125
  circle A320 centre (48.81, 40.08) radius 1.125
  circle A321 centre (51.35, 40.08) radius 1.125
  circle A322 centre (53.89, 40.08) radius 1.125
  circle A323 centre (56.43, 40.08) radius 1.125
  circle A324 centre (58.97, 40.08) radius 1.125
  circle A325 centre (61.51, 40.08) radius 1.125
  circle A326 centre (64.05, 40.08) radius 1.125
  circle A327 centre (66.59, 40.08) radius 1.125
  circle A328 centre (69.13, 40.08) radius 1.125
  circle A329 centre (71.67, 40.08) radius 1.125
  circle A330 centre (74.21, 40.08) radius 1.125
  circle A331 centre (76.75, 40.08) radius 1.125
  circle A332 centre (79.29, 40.08) radius 1.125
  circle A333 centre (81.83, 40.08) radius 1.125
  circle A334 centre (8.17, 37.54) radius 1.125
  circle A335 centre (10.71, 37.54) radius 1.125
  circle A336 centre (13.25, 37.54) radius 1.125
  circle A337 centre (15.79, 37.54) radius 1.125
  circle A338 centre (18.33, 37.54) radius 1.125
  circle A339 centre (20.87, 37.54) radius 1.125
  circle A340 centre (23.41, 37.54) radius 1.125
  circle A341 centre (25.95, 37.54) radius 1.125
  circle A342 centre (28.49, 37.54) radius 1.125
  circle A343 centre (31.03, 37.54) radius 1.125
  circle A344 centre (33.57, 37.54) radius 1.125
  circle A345 centre (36.11, 37.54) radius 1.125
  circle A346 centre (38.65, 37.54) radius 1.125
  circle A347 centre (41.19, 37.54) radius 1.125
  circle A348 centre (43.73, 37.54) radius 1.125
  circle A349 centre (46.27, 37.54) radius 1.125
  circle A350 centre (48.81, 37.54) radius 1.125
  circle A351 centre (51.35, 37.54) radius 1.125
  circle A352 centre (53.89, 37.54) radius 1.125
  circle A353 centre (56.43, 37.54) radius 1.125
  circle A354 centre (58.97, 37.54) radius 1.125
  circle A355 centre (61.51, 37.54) radius 1.125
  circle A356 centre (64.05, 37.54) radius 1.125
  circle A357 centre (66.59, 37.54) radius 1.125
  circle A358 centre (69.13, 37.54) radius 1.125
  circle A359 centre (71.67, 37.54) radius 1.125
  circle A360 centre (74.21, 37.54) radius 1.125
  circle A361 centre (76.75, 37.54) radius 1.125
  circle A362 centre (79.29, 37.54) radius 1.125
  circle A363 centre (81.83, 37.54) radius 1.125
  circle A364 centre (8.17, 35) radius 1.125
  circle A365 centre (10.71, 35) radius 1.125
  circle A366 centre (13.25, 35) radius 1.125
  circle A367 centre (15.79, 35) radius 1.125
  circle A368 centre (18.33, 35) radius 1.125
  circle A369 centre (20.87, 35) radius 1.125
  circle A370 centre (23.41, 35) radius 1.125
  circle A371 centre (25.95, 35) radius 1.125
  circle A372 centre (28.49, 35) radius 1.125
  circle A373 centre (31.03, 35) radius 1.125
  circle A374 centre (33.57, 35) radius 1.125
  circle A375 centre (36.11, 35) radius 1.125
  circle A376 centre (38.65, 35) radius 1.125
  circle A377 centre (41.19, 35) radius 1.125
  circle A378 centre (43.73, 35) radius 1.125
  circle A379 centre (46.27, 35) radius 1.125
  circle A380 centre (48.81, 35) radius 1.125
  circle A381 centre (51.35, 35) radius 1.125
  circle A382 centre (53.89, 35) radius 1.125
  circle A383 centre (56.43, 35) radius 1.125
  circle A384 centre (58.97, 35) radius 1.125
  circle A385 centre (61.51, 35) radius 1.125
  circle A386 centre (64.05, 35) radius 1.125
  circle A387 centre (66.59, 35) radius 1.125
  circle A388 centre (69.13, 35) radius 1.125
  circle A389 centre (71.67, 35) radius 1.125
  circle A390 centre (74.21, 35) radius 1.125
  circle A391 centre (76.75, 35) radius 1.125
  circle A392 centre (79.29, 35) radius 1.125
  circle A393 centre (81.83, 35) radius 1.125
  circle A394 centre (8.17, 32.46) radius 1.125
  circle A395 centre (10.71, 32.46) radius 1.125
  circle A396 centre (13.25, 32.46) radius 1.125
  circle A397 centre (15.79, 32.46) radius 1.125
  circle A398 centre (18.33, 32.46) radius 1.125
  circle A399 centre (20.87, 32.46) radius 1.125
  circle A400 centre (23.41, 32.46) radius 1.125
  circle A401 centre (25.95, 32.46) radius 1.125
  circle A402 centre (28.49, 32.46) radius 1.125
  circle A403 centre (31.03, 32.46) radius 1.125
  circle A404 centre (33.57, 32.46) radius 1.125
  circle A405 centre (36.11, 32.46) radius 1.125
  circle A406 centre (38.65, 32.46) radius 1.125
  circle A407 centre (41.19, 32.46) radius 1.125
  circle A408 centre (43.73, 32.46) radius 1.125
  circle A409 centre (46.27, 32.46) radius 1.125
  circle A410 centre (48.81, 32.46) radius 1.125
  circle A411 centre (51.35, 32.46) radius 1.125
  circle A412 centre (53.89, 32.46) radius 1.125
  circle A413 centre (56.43, 32.46) radius 1.125
  circle A414 centre (58.97, 32.46) radius 1.125
  circle A415 centre (61.51, 32.46) radius 1.125
  circle A416 centre (64.05, 32.46) radius 1.125
  circle A417 centre (66.59, 32.46) radius 1.125
  circle A418 centre (69.13, 32.46) radius 1.125
  circle A419 centre (71.67, 32.46) radius 1.125
  circle A420 centre (74.21, 32.46) radius 1.125
  circle A421 centre (76.75, 32.46) radius 1.125
  circle A422 centre (79.29, 32.46) radius 1.125
  circle A423 centre (81.83, 32.46) radius 1.125
  circle A424 centre (8.17, 29.92) radius 1.125
  circle A425 centre (10.71, 29.92) radius 1.125
  circle A426 centre (13.25, 29.92) radius 1.125
  circle A427 centre (15.79, 29.92) radius 1.125
  circle A428 centre (18.33, 29.92) radius 1.125
  circle A429 centre (20.87, 29.92) radius 1.125
  circle A430 centre (23.41, 29.92) radius 1.125
  circle A431 centre (25.95, 29.92) radius 1.125
  circle A432 centre (28.49, 29.92) radius 1.125
  circle A433 centre (31.03, 29.92) radius 1.125
  circle A434 centre (33.57, 29.92) radius 1.125
  circle A435 centre (36.11, 29.92) radius 1.125
  circle A436 centre (38.65, 29.92) radius 1.125
  circle A437 centre (41.19, 29.92) radius 1.125
  circle A438 centre (43.73, 29.92) radius 1.125
  circle A439 centre (46.27, 29.92) radius 1.125
  circle A440 centre (48.81, 29.92) radius 1.125
  circle A441 centre (51.35, 29.92) radius 1.125
  circle A442 centre (53.89, 29.92) radius 1.125
  circle A443 centre (56.43, 29.92) radius 1.125
  circle A444 centre (58.97, 29.92) radius 1.125
  circle A445 centre (61.51, 29.92) radius 1.125
  circle A446 centre (64.05, 29.92) radius 1.125
  circle A447 centre (66.59, 29.92) radius 1.125
  circle A448 centre (69.13, 29.92) radius 1.125
  circle A449 centre (71.67, 29.92) radius 1.125
  circle A450 centre (74.21, 29.92) radius 1.125
  circle A451 centre (76.75, 29.92) radius 1.125
  circle A452 centre (79.29, 29.92) radius 1.125
  circle A453 centre (81.83, 29.92) radius 1.125
  circle A454 centre (8.17, 27.38) radius 1.125
  circle A455 centre (10.71, 27.38) radius 1.125
  circle A456 centre (13.25, 27.38) radius 1.125
  circle A457 centre (15.79, 27.38) radius 1.125
  circle A458 centre (18.33, 27.38) radius 1.125
  circle A459 centre (20.87, 27.38) radius 1.125
  circle A460 centre (23.41, 27.38) radius 1.125
  circle A461 centre (25.95, 27.38) radius 1.125
  circle A462 centre (28.49, 27.38) radius 1.125
  circle A463 centre (31.03, 27.38) radius 1.125
  circle A464 centre (33.57, 27.38) radius 1.125
  circle A465 centre (36.11, 27.38) radius 1.125
  circle A466 centre (38.65, 27.38) radius 1.125
  circle A467 centre (41.19, 27.38) radius 1.125
  circle A468 centre (43.73, 27.38) radius 1.125
  circle A469 centre (46.27, 27.38) radius 1.125
  circle A470 centre (48.81, 27.38) radius 1.125
  circle A471 centre (51.35, 27.38) radius 1.125
  circle A472 centre (53.89, 27.38) radius 1.125
  circle A473 centre (56.43, 27.38) radius 1.125
  circle A474 centre (58.97, 27.38) radius 1.125
  circle A475 centre (61.51, 27.38) radius 1.125
  circle A476 centre (64.05, 27.38) radius 1.125
  circle A477 centre (66.59, 27.38) radius 1.125
  circle A478 centre (69.13, 27.38) radius 1.125
  circle A479 centre (71.67, 27.38) radius 1.125
  circle A480 centre (74.21, 27.38) radius 1.125
  circle A481 centre (76.75, 27.38) radius 1.125
  circle A482 centre (79.29, 27.38) radius 1.125
  circle A483 centre (81.83, 27.38) radius 1.125
  circle A484 centre (8.17, 24.84) radius 1.125
  circle A485 centre (10.71, 24.84) radius 1.125
  circle A486 centre (13.25, 24.84) radius 1.125
  circle A487 centre (15.79, 24.84) radius 1.125
  circle A488 centre (18.33, 24.84) radius 1.125
  circle A489 centre (20.87, 24.84) radius 1.125
  circle A490 centre (23.41, 24.84) radius 1.125
  circle A491 centre (25.95, 24.84) radius 1.125
  circle A492 centre (28.49, 24.84) radius 1.125
  circle A493 centre (31.03, 24.84) radius 1.125
  circle A494 centre (33.57, 24.84) radius 1.125
  circle A495 centre (36.11, 24.84) radius 1.125
  circle A496 centre (38.65, 24.84) radius 1.125
  circle A497 centre (41.19, 24.84) radius 1.125
  circle A498 centre (43.73, 24.84) radius 1.125
  circle A499 centre (46.27, 24.84) radius 1.125
  circle A500 centre (48.81, 24.84) radius 1.125
  circle A501 centre (51.35, 24.84) radius 1.125
  circle A502 centre (53.89, 24.84) radius 1.125
  circle A503 centre (56.43, 24.84) radius 1.125
  circle A504 centre (58.97, 24.84) radius 1.125
  circle A505 centre (61.51, 24.84) radius 1.125
  circle A506 centre (64.05, 24.84) radius 1.125
  circle A507 centre (66.59, 24.84) radius 1.125
  circle A508 centre (69.13, 24.84) radius 1.125
  circle A509 centre (71.67, 24.84) radius 1.125
  circle A510 centre (74.21, 24.84) radius 1.125
  circle A511 centre (76.75, 24.84) radius 1.125
  circle A512 centre (79.29, 24.84) radius 1.125
  circle A513 centre (81.83, 24.84) radius 1.125
  circle A514 centre (8.17, 22.3) radius 1.125
  circle A515 centre (10.71, 22.3) radius 1.125
  circle A516 centre (13.25, 22.3) radius 1.125
  circle A517 centre (15.79, 22.3) radius 1.125
  circle A518 centre (18.33, 22.3) radius 1.125
  circle A519 centre (20.87, 22.3) radius 1.125
  circle A520 centre (23.41, 22.3) radius 1.125
  circle A521 centre (25.95, 22.3) radius 1.125
  circle A522 centre (28.49, 22.3) radius 1.125
  circle A523 centre (31.03, 22.3) radius 1.125
  circle A524 centre (33.57, 22.3) radius 1.125
  circle A525 centre (36.11, 22.3) radius 1.125
  circle A526 centre (38.65, 22.3) radius 1.125
  circle A527 centre (41.19, 22.3) radius 1.125
  circle A528 centre (43.73, 22.3) radius 1.125
  circle A529 centre (46.27, 22.3) radius 1.125
  circle A530 centre (48.81, 22.3) radius 1.125
  circle A531 centre (51.35, 22.3) radius 1.125
  circle A532 centre (53.89, 22.3) radius 1.125
  circle A533 centre (56.43, 22.3) radius 1.125
  circle A534 centre (58.97, 22.3) radius 1.125
  circle A535 centre (61.51, 22.3) radius 1.125
  circle A536 centre (64.05, 22.3) radius 1.125
  circle A537 centre (66.59, 22.3) radius 1.125
  circle A538 centre (69.13, 22.3) radius 1.125
  circle A539 centre (71.67, 22.3) radius 1.125
  circle A540 centre (74.21, 22.3) radius 1.125
  circle A541 centre (76.75, 22.3) radius 1.125
  circle A542 centre (79.29, 22.3) radius 1.125